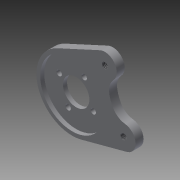
# Autodesk Inventor part: mount_plate
Saved by Autodesk Inventor 2015 (Build 190159000, 159)
## iProperties
Created: 2014-11-17
Part Number: mount_plate
Material: Generic
Document SubType Name: Modeling
Designer: brent
Density: 1 g/cm^3
Appearance: Default
Mass: 21.0965 g
Surface Area: 111.116 cm^2
Volume: 21.0965 cm^3
Author: brent
Autodesk Inventor part; units mm, degrees
ref_plane "YZ Plane" through (0, 0, 0) normal (1, 0, 0) x (0, 1, 0)
ref_plane "XZ Plane" through (0, 0, 0) normal (0, 1, 0) x (-1, 0, 0)
ref_plane "XY Plane" through (0, 0, 0) normal (0, 0, 1) x (1, 0, 0)
derived "mount_sketch.ipt"
sketch "Sketch2" plane through (0, 0, 0) normal (0, 0, 1) x (1, 0, 0)
  line L0 (72.4396, -72.2948) -> (-70.2441, 86.1715)
  line L1 (30.3736, -26.3701) -> (-42.626, -26.3701)
  circle A0 centre (-21.7992, 32.368) radius 3.9688
  circle A1 centre (-21.7992, 32.368) radius 9
  circle A2 centre (-82.0682, 4.3924) radius 2.15
  line L2 (-82.0682, 4.3924) -> (-108.234, 19.0673)
  circle A3 centre (-108.234, 19.0673) radius 2.15
  line L3 (-87.8136, 24.8127) -> (-102.4886, -1.353)
  circle A4 centre (-87.8136, 24.8127) radius 2.15
  circle A5 centre (-102.4886, -1.353) radius 2.15
  line L4 (-95.1511, 11.7299) -> (-21.7992, 32.368)
  line L5 (-86.579, -18.7372) -> (-13.227, 1.9009)
  line L6 (-103.7232, 42.1969) -> (-30.3713, 62.835)
  circle A6 centre (-95.1511, 11.7299) radius 10.5
  arc A7 (-103.7232, 42.1969) -> (-86.579, -18.7372) centre (-95.1511, 11.7299) ccw
  circle A8 centre (-21.7992, 32.368) radius 31.65
  line L7 (-13.663, 36.2154) -> (8.2274, 42.3744)
  line L8 (-12.8505, 33.3275) -> (9.0399, 39.4865)
  line L9 (-57.8777, 55.0959) -> (-30.3713, 62.835)
  line L10 (-40.7335, -5.8382) -> (-13.227, 1.9009)
  arc A9 (-52.4323, 6.082) -> (-61.6446, 38.8243) centre (-82.7333, 15.2237) ccw
  arc A10 (-57.8777, 55.0959) -> (-61.6446, 38.8243) centre (-55.298, 45.9269) ccw
  arc A11 (-52.4323, 6.082) -> (-40.7335, -5.8382) centre (-43.3132, 3.3308) ccw
  line L11 (-55.298, 45.9269) -> (-49.1853, 47.6467) construction
  line L12 (-54.6066, 43.4696) -> (-48.4939, 45.1894)
  line L13 (-49.8767, 50.104) -> (-55.9893, 48.3842)
  arc A12 (-55.9893, 48.3842) -> (-54.6066, 43.4696) centre (-55.298, 45.9269) ccw
  arc A13 (-48.4939, 45.1894) -> (-49.8767, 50.104) centre (-49.1853, 47.6467) ccw
  line L14 (-43.3132, 3.3308) -> (-37.2006, 5.0506) construction
  line L15 (-42.6219, 0.8735) -> (-36.5092, 2.5933)
  line L16 (-37.8919, 7.5079) -> (-44.0046, 5.7881)
  arc A14 (-44.0046, 5.7881) -> (-42.6219, 0.8735) centre (-43.3132, 3.3308) ccw
  arc A15 (-36.5092, 2.5933) -> (-37.8919, 7.5079) centre (-37.2006, 5.0506) ccw
  circle A16 centre (-52.2416, 46.7868) radius 2.413
  circle A17 centre (-40.2569, 4.1907) radius 2.413
  arc A18 (-37.6771, -4.9783) -> (-42.8367, 13.3597) centre (-40.2569, 4.1907) ccw
  arc A19 (-49.6619, 37.6178) -> (-54.8214, 55.9558) centre (-52.2416, 46.7868) ccw
  arc A20 (-49.6619, 37.6178) -> (-42.8367, 13.3597) centre (-21.7992, 32.368) ccw
  line L17 (-52.2416, 46.7868) -> (-40.2569, 4.1907)
  point P0 (0, 0)
  point P1 (-91.3054, 45.6908)
  point P2 (-74.1611, -15.2433)
  point P3 (-52.2416, 46.7868)
  point P4 (-40.2569, 4.1907)
extrude "Extrusion1" add sketch "Sketch2" along normal blind 6.35 contours L5 A11 A9 A8 L17 L16 A14 L15 A15 A18 | A8 A15 L16 L17 A18 | L5 A7 L6 A10 A9 A11 | A15 L15 A14 L16 L17 A17 A8 | A8 A17 L16 A15 | L17 A8 L4 A20 | L4 A8 L17 A20 | L17 A8 L12 A13 A19 | A8 L16 L17 | A8 A13 L13 A12 L12 L17 A9 A10 L6 A19 | L17 L12 A8 | A17 L17 L16 A8 | A13 L12 A8 A16 | A8 A16 L17 L12 A12 L13 A13 | L12 L17 A16 A8
fillet "Fillet1" radius 12.7 2 edges at (-49.6619, 37.6178, 3.175) (-42.8367, 13.3597, 3.175)
sketch "Sketch3" plane through (-95.1511, 11.7299, 6.35) normal (0, 0, 1) x (0.9626241, 0.2708411, 0)
  circle A0 centre (50.8006, -22.125) radius 2.413 projected
  circle A1 centre (50.8006, 22.125) radius 2.413 projected
  arc A2 (55.046, 13.5985) -> (50.8006, 31.65) centre (50.8006, 22.125) ccw projected
  line L0 (50.8006, 31.65) -> (0, 31.65) projected
  arc A3 (0, 31.65) -> (0, -31.65) centre (0, 0) ccw projected
  line L1 (0, -31.65) -> (50.8006, -31.65) projected
  arc A4 (50.8006, -31.65) -> (55.046, -13.5985) centre (50.8006, -22.125) ccw projected
  arc A5 (48.1362, -4.0389) -> (55.046, -13.5985) centre (60.7067, -2.2298) ccw projected
  arc A6 (48.1362, 4.0389) -> (48.1362, -4.0389) centre (76.2, 0) ccw projected
  arc A7 (55.046, 13.5985) -> (48.1362, 4.0389) centre (60.7067, 2.2298) ccw projected
  circle A8 centre (0, 0) radius 10.5 projected
  circle A9 centre (-10.6066, -10.6066) radius 2.15 projected
  circle A10 centre (10.6066, 10.6066) radius 2.15 projected
  circle A11 centre (-10.6066, 10.6066) radius 2.15 projected
  circle A12 centre (10.6066, -10.6066) radius 2.15 projected
  circle A13 centre (0, 0) radius 25.5
  circle A14 centre (0, 0) radius 28.5
  line L2 (50.8006, 31.65) -> (0, 31.65) projected
  line L3 (50.8006, 31.65) -> (-1.7343, 28.4472)
  line L4 (0, -31.65) -> (50.8006, -31.65) projected
  line L5 (50.8006, -31.65) -> (-1.7343, -28.4472)
  point P0 (88.4178, -37.0623)
  dimension "d4" = 51
  dimension "d5" = 3
  constraints: 4 end point, 2 centre point, 2 coincident, 2 point on circle, 2 tangent
  measures "d4" diameter of A13
  measures "d5" radial gap between concentric circles of A13 A14
extrude "Extrusion2" cut sketch "Sketch3" against normal through all contours L3 A14 L5 L1 A3 L0
extrude "Extrusion3" cut sketch "Sketch3" against normal blind 3.175 contours A13
thread "Thread1" size "10-32 UNF" class "2B" standard "ANSI Unified Screw Threads" full length
thread "Thread2" size "10-24 UNC" class "2B" standard "ANSI Unified Screw Threads" full length
body "Solid1"
